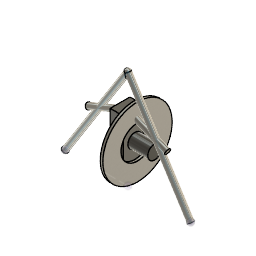
fs-suspension-corner-v1 (Autodesk Fusion 360 design; units mm, degrees)
part number: 2026-06-22-14-18-39-388
part number: 2026-06-22-14-23-19-592
part number: 2026-06-22-14-50-41-601
part number: 2026-06-22-15-43-07-512
part number: 2026-06-22-16-22-04-503
part number: 2026-06-22-16-33-34-143
Autodesk Fusion 360 part; units mm, degrees
sketch "Sketch1" plane through (0, 0, 0) normal (0, 0, 1) x (1, 0, 0) in component "Lower A-arm"
  line L0 (0, 0) -> (-190, 0) construction
  line L1 (0, 0) -> (190, 0) construction
  line L2 (-190, 0) -> (0, 300)
  line L3 (0, 300) -> (190, 0)
  dimension "d8" = 190
  dimension "d9" = 190
  dimension "d10" = 300
  constraint coincident L0.start L1.start
  constraint horizontal L0
  constraint parallel L0 L1
  measures "d8" distance of L0.start L0.end
  measures "d9" distance of L0.start L1.end
  measures "d10" distance of L0.start L2.end
ref_plane "WorkPlane1" through (190, 0, 0) normal (0.535052, -0.844819, 0) x (0.844819, 0.535052, 0) in component "Lower A-arm"
sketch "Sketch2" plane through (190, 0, 0) normal (0.535052, -0.844819, 0) x (0.844819, 0.535052, 0) in component "Lower A-arm"
  circle A0 centre (0, 0) radius 9
  dimension "d12" = 18
  constraint coincident A0.centre origin
  measures "d12" diameter of A0
sweep "Sweep1" add kept parallel profiles "Sketch2" path "Sketch1" along L3 section 1 makes body 1 in component "Lower A-arm"
ref_plane "WorkPlane2" through (-190, 0, 0) normal (0.535052, 0.844819, 0) x (-0.844819, 0.535052, 0) in component "Lower A-arm"
sketch "Sketch3" plane through (-190, 0, 0) normal (0.535052, 0.844819, 0) x (-0.844819, 0.535052, 0) in component "Lower A-arm"
  circle A0 centre (0, 0) radius 9
  dimension "d20" = 18
  constraint coincident A0.centre origin
  measures "d20" diameter of A0
sweep "Sweep2" add kept parallel profiles "Sketch3" path "Sketch1" along L2 section 1 bodies 1 in component "Lower A-arm"
sphere "SpherePrimitive1" add diameter 18 placed x (1, 0, 0) y (0, 1, 0) z (0, 0, 1) at (0, 300, 0) bodies 1 in component "Lower A-arm"
fillet "Fillet1" radius 1 1 edges at (0, 283.1792, 0) on bodies 1 in component "Lower A-arm"
fillet "Fillet1" radius 1 1 faces at (6.1308, 306.3044, -1.9151) on bodies 1 in component "Lower A-arm"
sketch "Sketch1 (2)" plane through (0, 0, 0) normal (0, 1, 0) x (1, 0, 0) in component "Upper A-arm"
  line L0 (0, 0) -> (-120, 0)
  line L1 (0, 0) -> (120, 0)
  line L2 (-120, 0) -> (0, -50)
  line L3 (0, -50) -> (120, 0)
  dimension "d32" = 120
  dimension "d33" = 120
  dimension "d34" = 50
  constraint coincident L0.start L1.start
  constraint horizontal L0
  constraint parallel L0 L1
  measures "d32" distance of L0.start L0.end
  measures "d33" distance of L0.start L1.end
  measures "d34" distance of L0.start L2.end
ref_plane "WorkPlane1" through (120, 0, 0) normal (0.923077, 0, -0.384615) x (0, 1, 0) in component "Upper A-arm"
sketch "Sketch2 (2)" plane through (120, 0, 0) normal (0.923077, 0, -0.384615) x (0, 1, 0) in component "Upper A-arm"
  circle A0 centre (0, 0) radius 9
  dimension "d36" = 18
  constraint coincident A0.centre origin
  measures "d36" diameter of A0
sweep "Sweep1'" add kept parallel profiles "Sketch2 (2)" path "Sketch1 (2)" along L3 section 1 separate body makes body 2 in component "Upper A-arm"
ref_plane "WorkPlane2" through (-120, 0, 0) normal (0.923077, 0, 0.384615) x (0, 1, 0) in component "Upper A-arm"
sketch "Sketch3 (2)" plane through (-120, 0, 0) normal (0.923077, 0, 0.384615) x (0, 1, 0) in component "Upper A-arm"
  circle A0 centre (0, 0) radius 9
  dimension "d44" = 18
  constraint coincident A0.centre origin
  measures "d44" diameter of A0
sweep "Sweep2'" add kept parallel profiles "Sketch3 (2)" path "Sketch1 (2)" along L2 section 1 bodies 2 in component "Upper A-arm"
sphere "SpherePrimitive1'" add diameter 18 placed x (1, 0, 0) y (0, 1, 0) z (0, 0, 1) at (-35, -15, 0) separate body makes body 3 in component "Upper A-arm"
delete_face "DeleteFace1" 1 faces at (-26.4673, -12.8726, -1.9151) on bodies 3 in component "Upper A-arm"
sphere "SpherePrimitive2" add diameter 18 placed x (1, 0, 0) y (0, 0, -1) z (0, 1, 0) at (0, 0, 50) bodies 2 in component "Upper A-arm"
move_body "Move1" bodies 2 to x (1, 0, 0) y (0, 1, 0) z (0, 0, 1) at (0, 0, 150) in component "Upper A-arm"
sketch "Sketch1 (3)" plane through (0, 0, 0) normal (1, 0, 0) x (0, 1, 0) in component "Upright"
  line L0 (0, 0) -> (-60, 0)
  line L1 (-60, 0) -> (-60, 150)
  line L2 (-60, 150) -> (0, 150)
  line L3 (0, 150) -> (0, 0)
  dimension "d53" = 60
  dimension "d54" = 150
  constraint horizontal L0
  constraint vertical L1
  constraint horizontal L2
  constraint vertical L3
  constraint coincident L0.start L3.end
  measures "d53" distance of L0.start L0.end
  measures "d54" distance of L0.start L2.end
extrude "Extrude1" add sketch "Sketch1 (3)" along normal blind 40 separate body makes body 4 in component "Upright"
move_body "Move1'" bodies 4 to x (1, 0, 0) y (0, 1, 0) z (0, 0, 1) at (-19.1518, -125, 11.4911) in component "Upright"
sketch "Sketch2 (3)" plane through (20.8482, 0, 0) normal (1, 0, 0) x (0, 1, 0) in component "Upright"
  line L0 (-125, 161.4911) -> (-185, 161.4911)
  line L1 (-185, 161.4911) -> (-185, 11.4911)
  line L2 (-185, 11.4911) -> (-125, 11.4911)
  line L3 (-125, 11.4911) -> (-125, 161.4911)
  circle A0 centre (-150, 80) radius 21
  dimension "d57" = 42
  measures "d57" diameter of A0
extrude "Extrude2" cut sketch "Sketch2 (3)" against normal blind 40 contours A0 bodies 4 in component "Upright"
sketch "Sketch1 (4)" plane through (20.8482, 0, 0) normal (1, 0, 0) x (0, 1, 0) in component "Hub"
  circle A0 centre (0, 130) radius 21
  line L0 (25, 211.4911) -> (-35, 211.4911)
  line L1 (-35, 211.4911) -> (-35, 61.4911)
  line L2 (-35, 61.4911) -> (25, 61.4911)
  line L3 (25, 61.4911) -> (25, 211.4911)
  circle A1 centre (0, 130) radius 21
  circle A2 centre (0, 130) radius 21
  circle A3 centre (0, 130) radius 50
  dimension "d60" = 100
  constraint concentric A1 A2
  constraint concentric A1 A3
  measures "d60" diameter of A3
extrude "Extrude1'" add sketch "Sketch1 (4)" along normal blind 60 separate body contours A0 A1 A2 makes body 5 in component "Hub"
extrude "Extrude2'" add sketch "Sketch1 (4)" against normal blind 15 separate body contours L3 A3 | L1 A3 makes body 6 at (10.8482, 48.4539, 142.3379) makes body 7 at (10.8482, -48.2529, 143.1019) in component "Hub"
sketch "Sketch1 (5)" plane through (20.8482, 0, 0) normal (1, 0, 0) x (0, 1, 0) in component "Brake-disc"
  circle A0 centre (0, 130) radius 50
  circle A1 centre (0, 130) radius 40
  circle A2 centre (0, 130) radius 105
  dimension "d65" = 80
  dimension "d66" = 210
  constraint concentric A0 A1
  constraint concentric A1 A2
  measures "d65" diameter of A1
  measures "d66" diameter of A2
extrude "Extrude1''" add sketch "Sketch1 (5)" along normal blind 8 separate body contours A2 makes body 8 in component "Brake-disc"
component "Upper A-arm" placed x (1, 0, 0) y (0, 1, 0) z (0, 0, 1) at (0, 0, 0)
component "Upright" placed x (1, 0, 0) y (0, 1, 0) z (0, 0, 1) at (0, 150, 50)
component "Lower A-arm" placed x (1, 0, 0) y (0, 0, 1) z (0, -1, 0) at (0, 0, 0)
component "Hub" placed x (1, 0, 0) y (0, 1, 0) z (0, 0, 1) at (0, 0, 0)
component "Brake-disc" placed x (1, 0, 0) y (0, 1, 0) z (0, 0, 1) at (0, 0, 0)
equation "chassis_spread = 380 mm"
equation "tube_od = 18 mm"
equation "wall_thickness = 1.5 mm"
equation "lower_wishbone_length = 300 mm"
equation "upper_wishbone_length = 240 mm"
equation "d8 = chassis_spread / 2"
equation "d9 = chassis_spread / 2"
equation "d10 = lower_wishbone_length"
equation "d12 = tube_od"
equation "d20 = tube_od"
equation "d27 = tube_od"
equation "d32 = upper_wishbone_length / 2"
equation "d33 = upper_wishbone_length / 2"
equation "d36 = tube_od"
equation "d44 = tube_od"
